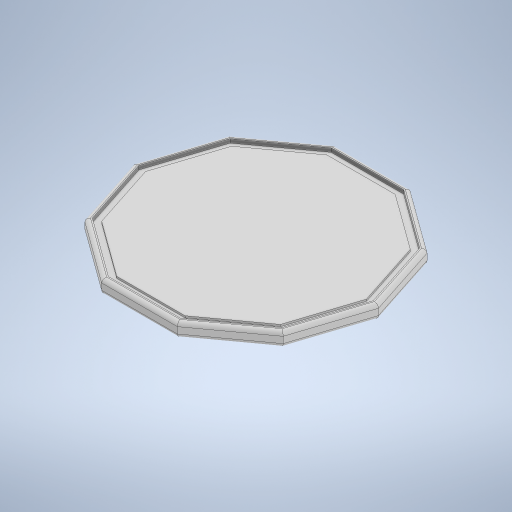
# Autodesk Inventor part: OV-PAM_n_10_bottom
Saved by Autodesk Inventor 2024 (Build 280153000, 153)
## iProperties
Created: 2023-08-31
Part Number: OV-PAM_n_10_bottom
Material: 일반
Document SubType Name: Modeling
Designer: jsw
Density: 1 g/cm^3
Appearance: 기본값
Author: jsw
Autodesk Inventor part; units mm, degrees
ref_plane "YZ Plane" through (0, 0, 0) normal (1, 0, 0) x (0, 1, 0)
ref_plane "XZ Plane" through (0, 0, 0) normal (0, 1, 0) x (-1, 0, 0)
ref_plane "XY Plane" through (0, 0, 0) normal (0, 0, 1) x (1, 0, 0)
sketch "스케치1" plane through (0, 0, 0) normal (0, 1, 0) x (-1, 0, 0)
  line L0 (-10.9012, 33.5504) -> (10.9012, 33.5504)
  line L1 (10.9012, 33.5504) -> (28.5397, 20.7353)
  line L2 (28.5397, 20.7353) -> (35.277, 0)
  line L3 (35.277, 0) -> (28.5397, -20.7353)
  line L4 (28.5397, -20.7353) -> (10.9012, -33.5504)
  line L5 (10.9012, -33.5504) -> (-10.9012, -33.5504)
  line L6 (-10.9012, -33.5504) -> (-28.5397, -20.7353)
  line L7 (-28.5397, -20.7353) -> (-35.277, 0)
  line L8 (-35.277, 0) -> (-28.5397, 20.7353)
  line L9 (-28.5397, 20.7353) -> (-10.9012, 33.5504)
  line L10 (11.9409, -36.7504) -> (-11.9409, -36.7504)
  line L11 (-11.9409, -36.7504) -> (-31.2618, -22.713)
  line L12 (-31.2618, -22.713) -> (-38.6417, 0)
  line L13 (-38.6417, 0) -> (-31.2618, 22.713)
  line L14 (-31.2618, 22.713) -> (-11.9409, 36.7504)
  line L15 (-11.9409, 36.7504) -> (11.9409, 36.7504)
  line L16 (11.9409, 36.7504) -> (31.2618, 22.713)
  line L17 (31.2618, 22.713) -> (38.6417, 0)
  line L18 (38.6417, 0) -> (31.2618, -22.713)
  line L19 (31.2618, -22.713) -> (11.9409, -36.7504)
  point P0 (0, 0)
  point P1 (0, 0)
  point P2 (0, 0)
  dimension "d0" = 70.554
  dimension "d1" = 3.2
  constraints: 40 end point, 2 coincident, 2 horizontal, 42 other
  measures "d0" distance of L7.end L2.end
  measures "d1" distance between parallel lines of L3 L18
extrude "돌출1" add sketch "스케치1" along normal blind 4.4 contours L0 L1 L2 L3 L4 L5 L6 L7 L8 L9 | L10 L11 L12 L13 L14 L15 L16 L17 L18 L19
sketch "스케치2" plane through (0, 4.4, 0) normal (0, 1, 0) x (1, 0, 0)
  line L0 (-11.4211, 35.1504) -> (11.4211, 35.1504)
  line L1 (11.4211, 35.1504) -> (29.9007, 21.7242)
  line L2 (29.9007, 21.7242) -> (36.9593, 0)
  line L3 (36.9593, 0) -> (29.9007, -21.7242)
  line L4 (29.9007, -21.7242) -> (11.4211, -35.1504)
  line L5 (11.4211, -35.1504) -> (-11.4211, -35.1504)
  line L6 (-11.4211, -35.1504) -> (-29.9007, -21.7242)
  line L7 (-29.9007, -21.7242) -> (-36.9593, 0)
  line L8 (-36.9593, 0) -> (-29.9007, 21.7242)
  line L9 (-29.9007, 21.7242) -> (-11.4211, 35.1504)
  line L10 (-31.2618, 22.713) -> (-38.6417, 0) projected
  point P0 (0, 0)
  point P1 (0, 0)
  dimension "d4" = 1.6
  constraints: 20 end point, 1 coincident, 1 horizontal, 21 other
  measures "d4" distance between parallel lines of L8 L10
extrude "돌출2" cut sketch "스케치2" against normal blind 1.2
sketch "스케치3" plane through (0, 3.2, 0) normal (0, 1, 0) x (1, 0, 0)
  line L0 (-10.7712, 33.1504) -> (10.7712, 33.1504)
  line L1 (10.7712, 33.1504) -> (28.1994, 20.4881)
  line L2 (28.1994, 20.4881) -> (34.8564, 0)
  line L3 (34.8564, 0) -> (28.1994, -20.4881)
  line L4 (28.1994, -20.4881) -> (10.7712, -33.1504)
  line L5 (10.7712, -33.1504) -> (-10.7712, -33.1504)
  line L6 (-10.7712, -33.1504) -> (-28.1994, -20.4881)
  line L7 (-28.1994, -20.4881) -> (-34.8564, 0)
  line L8 (-34.8564, 0) -> (-28.1994, 20.4881)
  line L9 (-28.1994, 20.4881) -> (-10.7712, 33.1504)
  line L10 (-29.9007, 21.7242) -> (-11.4211, 35.1504) projected
  point P0 (0, 0)
  point P1 (0, 0)
  dimension "d7" = 2
  constraints: 20 end point, 1 coincident, 1 horizontal, 21 other
  measures "d7" distance between parallel lines of L10 L9
extrude "돌출3" add sketch "스케치3" along normal blind 0.6
fillet "모깎기1" radius 1.2 20 edges at (0, 4.4, 36.7504) (0, 0, 36.7504) (-21.6014, 4.4, 29.7317) (-21.6014, 0, 29.7317) (-34.9517, 4.4, 11.3565) (-34.9517, 4.4, -11.3565) (-21.6014, 4.4, -29.7317) (0, 4.4, -36.7504) (21.6014, 4.4, -29.7317) (34.9517, 4.4, -11.3565) (34.9517, 4.4, 11.3565) (21.6014, 4.4, 29.7317) (21.6014, 0, -29.7317) (0, 0, -36.7504) (-21.6014, 0, -29.7317) (-34.9517, 0, -11.3565) (-34.9517, 0, 11.3565) (34.9517, 0, -11.3565) (34.9517, 0, 11.3565) (21.6014, 0, 29.7317)
sketch "스케치6" plane through (0, 0, 0) normal (0, -1, 0) x (1, 0, 0)
  circle A0 centre (0, 0) radius 3.9688
  dimension "d26" = 7.9375
  constraints: 1 centre point, 1 coincident
  measures "d26" diameter of A0
extrude "돌출6" add sketch "스케치6" along normal blind 7.62
thread "스레드1" size "5/16-18 UNC" class "2A" standard "ANSI Unified Screw Threads" full length
sketch "스케치8" plane through (0, -7.62, 0) normal (-1, 0, 0) x (0, 0, 1)
  line L0 (3.9688, 0) -> (3.9688, 7.62)
  line L1 (3.9688, 7.62) -> (2.9225, 7.62)
  line L2 (2.9225, 7.62) -> (2.9225, 0)
  line L3 (2.9225, 0) -> (3.9688, 0)
  line L4 (0, -4.2505) -> (0, 14.7318) projected
  constraints: 8 end point
revolve "회전1" cut sketch "스케치8" angle 360 about axis through (0, -7.62, 0) along (0, 1, 0)
sketch "스케치9" plane through (0, -7.62, 0) normal (-1, 0, 0) x (0, 0, 1)
  line L0 (3.9688, 0) -> (3.9688, 7.62)
  line L1 (3.9688, 7.62) -> (2.9225, 7.62)
  line L2 (2.9225, 7.62) -> (2.9225, 0)
  line L3 (2.9225, 0) -> (3.9688, 0)
  line L4 (0, -4.2505) -> (0, 14.7318) projected
  constraints: 8 end point
revolve "회전2" add sketch "스케치9" angle 360 about axis through (0, -7.62, 0) along (0, 1, 0) separate body
sketch "스케치7" plane through (0, -7.62, 0) normal (1, 0, 0) x (0, 1, 0)
  line L0 (-0.8233, -2.994) -> (-0.7057, -2.994) construction
  line L1 (0.1175, -3.8976) -> (-0.0001, -4.1235) construction
  line L2 (-1.4112, -4.1235) -> (-1.5288, -3.8976) construction
  line L3 (-0.5881, -2.994) -> (-0.7057, -2.7681) construction
  line L4 (-0.7057, -2.7681) -> (-0.8233, -2.994) construction
  line L5 (-1.4112, -4.1235) -> (-1.2936, -3.8976) construction
  line L6 (-0.5881, -2.994) -> (-0.1177, -3.8976)
  line L7 (-1.5288, -3.8976) -> (-1.2936, -3.8976) construction
  arc A0 (-1.5288, -3.8976) -> (-1.4112, -3.9689) centre (-1.4112, -3.8363) ccw construction
  line L8 (0.1175, -3.8976) -> (-0.1177, -3.8976) construction
  line L9 (-1.4112, -4.1235) -> (-1.4112, -3.8976) construction
  line L10 (-0.0001, -4.1235) -> (-0.0001, -3.8976) construction
  line L11 (-0.7057, -2.7681) -> (-0.7057, -2.9226) construction
  line L12 (-1.4112, -3.9689) -> (-0.0001, -3.9689)
  arc A1 (-1.4112, -3.9689) -> (-1.2936, -3.8976) centre (-1.4112, -3.8363) ccw
  line L13 (-0.1177, -3.8976) -> (-0.0001, -4.1235) construction
  line L14 (-1.2936, -3.8976) -> (-0.8233, -2.994)
  line L15 (-0.0001, -0.0002) -> (-0.0001, 0.0177)
  line L16 (-0.0001, 0.0177) -> (-0.0001, -0.0002)
  line L17 (-0.0001, -0.0002) -> (0.0334, -0.0002)
  arc A2 (-0.1177, -3.8976) -> (-0.0001, -3.9689) centre (-0.0001, -3.8363) ccw
  arc A3 (-0.0001, -3.9689) -> (0.1175, -3.8976) centre (-0.0001, -3.8363) ccw construction
  arc A4 (-0.7057, -2.9226) -> (-0.8233, -2.994) centre (-0.7057, -3.0552) ccw
  arc A5 (-0.5881, -2.994) -> (-0.7057, -2.9226) centre (-0.7057, -3.0552) ccw
  line L18 (-0.7057, -2.9226) -> (-0.7057, -2.994) construction
  line L19 (-0.7057, -2.994) -> (-0.5881, -2.994) construction
  dimension "d31" = 55
  dimension "d32" = 0.2259
  dimension "d33" = 0.2259
  dimension "d36" = 1.4111
  constraints: 40 end point, 12 point on circle, 10 parallel, 8 tangent, 7 collinear, 6 centre point, 2 midpoint, 2 point on line, 1 horizontal, 1 perpendicular, 5 other
  measures "d31" angle of L6 L14
  measures "d32" distance of L3.end L0.end
  measures "d33" distance of L1.end L10.end
  measures "d36" distance from line of L1.end L9
coil "코일1" sketch "스케치7" operation cut axis through (0, -7.62, 0) along (0, 1, 0) pitch 1.4125 turns 7.392607 hand right bodies 2
equation "\"d31\" = d38"
equation "\"d38\" = 55deg"
